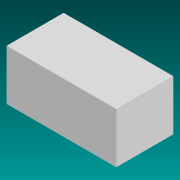
# Autodesk Inventor part: kleinere microswitch
Saved by Autodesk Inventor 2020 (Build 240168000, 168)
## iProperties
Created: 2020-05-29
Part Number: kleinere microswitch
Material: Generic
Document SubType Name: Modeling
Designer: stefa
Density: 1 g/cm^3
Appearance: Default
Author: stefa
Autodesk Inventor part; units mm, degrees
ref_plane "YZ Plane" through (0, 0, 0) normal (1, 0, 0) x (0, 1, 0)
ref_plane "XZ Plane" through (0, 0, 0) normal (0, 1, 0) x (-1, 0, 0)
ref_plane "XY Plane" through (0, 0, 0) normal (0, 0, 1) x (1, 0, 0)
sketch "Sketch1" plane through (0, 0, 0) normal (0, 0, 1) x (1, 0, 0)
  line L0 (-6.45, -2.95) -> (6.45, -2.95)
  line L1 (6.45, -2.95) -> (6.45, 2.95)
  line L2 (6.45, 2.95) -> (-6.45, 2.95)
  line L3 (-6.45, 2.95) -> (-6.45, -2.95)
  line L4 (-6.45, -2.95) -> (6.45, 2.95) construction
  line L5 (6.45, -2.95) -> (-6.45, 2.95) construction
  point P0 (0, 0)
  dimension "d0" = 12.9
  dimension "d1" = 5.9
  constraints: 12 end point, 2 midpoint, 2 parallel, 1 horizontal, 1 perpendicular
  measures "d0" distance of L2.end L1.end
  measures "d1" distance of L1.end L0.end
extrude "Extrusion1" add sketch "Sketch1" along normal blind 6.7
body "Solid1"
